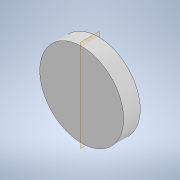
# Autodesk Inventor part: capFor6inchSch40Pipe
Saved by Autodesk Inventor 2021.1 (Build 251245000, 245)
## iProperties
Created: 2020-09-22
Part Number: capFor6inchSch40Pipe
Material: Generic
Document SubType Name: Modeling
Designer: robst
Density: 1 g/cm^3
Appearance: Default
Author: robst
Autodesk Inventor part; units mm, degrees
ref_plane "XZ Plane" through (0, 0, 0) normal (0, 1, 0) x (-1, 0, 0)
ref_plane "XY Plane" through (0, 0, 0) normal (0, 0, 1) x (1, 0, 0)
sketch "Sketch1" plane through (0, 0, 0) normal (0, 0, 1) x (1, 0, 0)
  circle A0 centre (0, 0) radius 87.3125
  circle A1 centre (0, 0) radius 92.075
  dimension "d0" = 174.625
  dimension "d1" = 4.7625
  constraints: 2 centre point, 2 coincident
  measures "d0" diameter of A0
  measures "d1" radial gap between concentric circles of A1 A0
extrude "Extrusion1" add sketch "Sketch1" along normal blind 4.7625 contours A0 | A1
extrude "Extrusion2" add sketch "Sketch1" against normal blind 31.75
sketch "Sketch2" plane through (0, 0, 0) normal (0, 0, -1) x (-1, 0, 0)
  line L0 (-80.4209, 0) -> (87.3125, 0) construction
  circle A0 centre (0, 0) radius 87.3125 construction
  spline S0 degree 2 poles (-73.9352, 1.1002) (-74.8615, 1.1002) (-76.4284, 1.7254) (-76.9996, 2.3506) knots 0 0 0 1 2 2 2
  spline S1 degree 2 poles (-76.9996, 2.3506) (-77.5708, 2.9681) (-78.196, 4.8206) (-78.196, 6.0248) knots 0 0 0 1 2 2 2
  spline S2 degree 2 poles (-78.196, 6.0248) (-78.196, 7.2212) (-77.5862, 8.9965) (-77.0073, 9.6526) knots 0 0 0 1 2 2 2
  spline S3 degree 2 poles (-77.0073, 9.6526) (-76.4361, 10.2933) (-74.8769, 10.9648) (-73.912, 10.9648) knots 0 0 0 1 2 2 2
  spline S4 degree 2 poles (-73.912, 10.9648) (-73.4335, 10.9648) (-72.5921, 10.8259) (-72.2371, 10.7178) knots 0 0 0 1 2 2 2
  spline S5 degree 2 poles (-72.2371, 10.7178) (-71.9283, 10.6175) (-71.2876, 10.3319) (-70.9712, 10.1621) knots 0 0 0 1 2 2 2
  line L1 (-70.9712, 10.1621) -> (-70.9712, 8.6337)
  line L2 (-70.9712, 8.6337) -> (-71.0715, 8.6337)
  spline S6 degree 2 poles (-71.0715, 8.6337) (-71.2413, 8.7881) (-71.7662, 9.2204) (-72.1444, 9.4288) knots 0 0 0 1 2 2 2
  spline S7 degree 2 poles (-72.1444, 9.4288) (-72.5072, 9.6295) (-73.364, 9.8842) (-73.9198, 9.8842) knots 0 0 0 1 2 2 2
  spline S8 degree 2 poles (-73.9198, 9.8842) (-74.5295, 9.8842) (-75.6179, 9.3825) (-76.027, 8.9039) knots 0 0 0 1 2 2 2
  spline S9 degree 2 poles (-76.027, 8.9039) (-76.4284, 8.4176) (-76.8761, 6.9433) (-76.8761, 6.0248) knots 0 0 0 1 2 2 2
  spline S10 degree 2 poles (-76.8761, 6.0248) (-76.8761, 5.0445) (-76.4052, 3.632) (-75.9961, 3.1457) knots 0 0 0 1 2 2 2
  spline S11 degree 2 poles (-75.9961, 3.1457) (-75.5947, 2.6748) (-74.5218, 2.1963) (-73.9198, 2.1963) knots 0 0 0 1 2 2 2
  spline S12 degree 2 poles (-73.9198, 2.1963) (-73.3717, 2.1963) (-72.4377, 2.4664) (-72.075, 2.6671) knots 0 0 0 1 2 2 2
  spline S13 degree 2 poles (-72.075, 2.6671) (-71.7276, 2.8678) (-71.2105, 3.2846) (-71.0638, 3.4313) knots 0 0 0 1 2 2 2
  line L3 (-71.0638, 3.4313) -> (-70.9712, 3.4313)
  line L4 (-70.9712, 3.4313) -> (-70.9712, 1.9184)
  spline S14 degree 2 poles (-70.9712, 1.9184) (-71.2876, 1.7717) (-71.8434, 1.5016) (-72.2371, 1.3781) knots 0 0 0 1 2 2 2
  spline S15 degree 2 poles (-72.2371, 1.3781) (-72.6539, 1.2391) (-73.364, 1.1002) (-73.9352, 1.1002) knots 0 0 0 1 2 2 2
  spline S16 degree 2 poles (-65.8999, 2.0264) (-66.0466, 1.9184) (-66.5406, 1.5324) (-66.7721, 1.4167) knots 0 0 0 1 2 2 2
  spline S17 degree 2 poles (-66.7721, 1.4167) (-67.0886, 1.2468) (-67.683, 1.0693) (-68.2233, 1.0693) knots 0 0 0 1 2 2 2
  spline S18 degree 2 poles (-68.2233, 1.0693) (-68.6633, 1.0693) (-69.4583, 1.4012) (-69.7593, 1.7023) knots 0 0 0 1 2 2 2
  spline S19 degree 2 poles (-69.7593, 1.7023) (-70.0449, 1.9956) (-70.3923, 2.8601) (-70.3923, 3.3386) knots 0 0 0 1 2 2 2
  spline S20 degree 2 poles (-70.3923, 3.3386) (-70.3923, 4.0796) (-69.767, 5.1294) (-69.0878, 5.4304) knots 0 0 0 1 2 2 2
  spline S21 degree 2 poles (-69.0878, 5.4304) (-68.4857, 5.7083) (-66.8493, 5.9167) (-65.8999, 5.9707) knots 0 0 0 1 2 2 2
  line L5 (-65.8999, 5.9707) -> (-65.8999, 6.2023)
  spline S22 degree 2 poles (-65.8999, 6.2023) (-65.8999, 6.6191) (-66.1546, 7.1363) (-66.3862, 7.2829) knots 0 0 0 1 2 2 2
  spline S23 degree 2 poles (-66.3862, 7.2829) (-66.6178, 7.4296) (-67.2816, 7.5222) (-67.6367, 7.5222) knots 0 0 0 1 2 2 2
  spline S24 degree 2 poles (-67.6367, 7.5222) (-68.0535, 7.5222) (-69.1804, 7.2752) (-69.7439, 7.0359) knots 0 0 0 1 2 2 2
  line L6 (-69.7439, 7.0359) -> (-69.8134, 7.0359)
  line L7 (-69.8134, 7.0359) -> (-69.8134, 8.2632)
  spline S25 degree 2 poles (-69.8134, 8.2632) (-69.4814, 8.3559) (-68.2387, 8.5874) (-67.6289, 8.5874) knots 0 0 0 1 2 2 2
  spline S26 degree 2 poles (-67.6289, 8.5874) (-66.8879, 8.5874) (-65.8768, 8.3559) (-65.4754, 8.0548) knots 0 0 0 1 2 2 2
  spline S27 degree 2 poles (-65.4754, 8.0548) (-65.0817, 7.7615) (-64.6958, 6.8275) (-64.6958, 6.156) knots 0 0 0 1 2 2 2
  line L8 (-64.6958, 6.156) -> (-64.6958, 1.27)
  line L9 (-64.6958, 1.27) -> (-65.8999, 1.27)
  line L10 (-65.8999, 1.27) -> (-65.8999, 2.0264)
  line L11 (-65.8999, 3.0299) -> (-65.8999, 5.0136)
  spline S28 degree 2 poles (-65.8999, 5.0136) (-66.3322, 4.975) (-67.6367, 4.8438) (-68.0458, 4.7203) knots 0 0 0 1 2 2 2
  spline S29 degree 2 poles (-68.0458, 4.7203) (-68.5243, 4.5736) (-69.1495, 3.9639) (-69.1495, 3.4235) knots 0 0 0 1 2 2 2
  spline S30 degree 2 poles (-69.1495, 3.4235) (-69.1495, 2.806) (-68.4548, 2.1808) (-67.791, 2.1808) knots 0 0 0 1 2 2 2
  spline S31 degree 2 poles (-67.791, 2.1808) (-67.2276, 2.1808) (-66.3013, 2.6671) (-65.8999, 3.0299) knots 0 0 0 1 2 2 2
  spline S32 degree 2 poles (-57.0156, 5.0368) (-57.0156, 3.246) (-58.7214, 1.1311) (-60.0259, 1.1311) knots 0 0 0 1 2 2 2
  spline S33 degree 2 poles (-60.0259, 1.1311) (-60.5585, 1.1311) (-61.3767, 1.3781) (-61.8012, 1.6328) knots 0 0 0 1 2 2 2
  line L12 (-61.8012, 1.6328) -> (-61.8012, -1.3621)
  line L13 (-61.8012, -1.3621) -> (-63.0054, -1.3621)
  line L14 (-63.0054, -1.3621) -> (-63.0054, 8.4176)
  line L15 (-63.0054, 8.4176) -> (-61.8012, 8.4176)
  line L16 (-61.8012, 8.4176) -> (-61.8012, 7.6689)
  spline S34 degree 2 poles (-61.8012, 7.6689) (-61.3536, 8.078) (-60.2575, 8.6183) (-59.6168, 8.6183) knots 0 0 0 1 2 2 2
  spline S35 degree 2 poles (-59.6168, 8.6183) (-58.3895, 8.6183) (-57.0156, 6.6732) (-57.0156, 5.0368) knots 0 0 0 1 2 2 2
  spline S36 degree 2 poles (-58.2583, 4.8978) (-58.2583, 6.1251) (-59.0379, 7.4759) (-59.9101, 7.4759) knots 0 0 0 1 2 2 2
  spline S37 degree 2 poles (-59.9101, 7.4759) (-60.4196, 7.4759) (-61.3767, 7.0205) (-61.8012, 6.6654) knots 0 0 0 1 2 2 2
  line L17 (-61.8012, 6.6654) -> (-61.8012, 2.6054)
  spline S38 degree 2 poles (-61.8012, 2.6054) (-61.3304, 2.3815) (-60.6589, 2.2117) (-60.2266, 2.2117) knots 0 0 0 1 2 2 2
  spline S39 degree 2 poles (-60.2266, 2.2117) (-59.2926, 2.2117) (-58.2583, 3.5856) (-58.2583, 4.8978) knots 0 0 0 1 2 2 2
  line L18 (-45.8851, 9.6681) -> (-50.3157, 9.6681)
  line L19 (-50.3157, 9.6681) -> (-50.3157, 6.9819)
  line L20 (-50.3157, 6.9819) -> (-46.0703, 6.9819)
  line L21 (-46.0703, 6.9819) -> (-46.0703, 5.855)
  line L22 (-46.0703, 5.855) -> (-50.3157, 5.855)
  line L23 (-50.3157, 5.855) -> (-50.3157, 1.27)
  line L24 (-50.3157, 1.27) -> (-51.5816, 1.27)
  line L25 (-51.5816, 1.27) -> (-51.5816, 10.795)
  line L26 (-51.5816, 10.795) -> (-45.8851, 10.795)
  line L27 (-45.8851, 10.795) -> (-45.8851, 9.6681)
  spline S40 degree 2 poles (-38.969, 4.8438) (-38.969, 3.0376) (-40.7058, 1.0693) (-42.1569, 1.0693) knots 0 0 0 1 2 2 2
  spline S41 degree 2 poles (-42.1569, 1.0693) (-43.6466, 1.0693) (-45.3525, 3.0994) (-45.3525, 4.8438) knots 0 0 0 1 2 2 2
  spline S42 degree 2 poles (-45.3525, 4.8438) (-45.3525, 6.6346) (-43.5926, 8.6183) (-42.1569, 8.6183) knots 0 0 0 1 2 2 2
  spline S43 degree 2 poles (-42.1569, 8.6183) (-40.7058, 8.6183) (-38.969, 6.6423) (-38.969, 4.8438) knots 0 0 0 1 2 2 2
  spline S44 degree 2 poles (-40.2118, 4.8438) (-40.2118, 6.2332) (-41.2229, 7.584) (-42.1569, 7.584) knots 0 0 0 1 2 2 2
  spline S45 degree 2 poles (-42.1569, 7.584) (-43.0909, 7.584) (-44.1098, 6.2332) (-44.1098, 4.8438) knots 0 0 0 1 2 2 2
  spline S46 degree 2 poles (-44.1098, 4.8438) (-44.1098, 3.493) (-43.0909, 2.1036) (-42.1569, 2.1036) knots 0 0 0 1 2 2 2
  spline S47 degree 2 poles (-42.1569, 2.1036) (-41.2306, 2.1036) (-40.2118, 3.4699) (-40.2118, 4.8438) knots 0 0 0 1 2 2 2
  line L28 (-33.9441, 7.1286) -> (-34.0058, 7.1286)
  spline S48 degree 2 poles (-34.0058, 7.1286) (-34.1448, 7.1672) (-34.4458, 7.1826) (-34.6542, 7.1826) knots 0 0 0 1 2 2 2
  spline S49 degree 2 poles (-34.6542, 7.1826) (-35.1405, 7.1826) (-36.0976, 6.7581) (-36.5299, 6.3413) knots 0 0 0 1 2 2 2
  line L29 (-36.5299, 6.3413) -> (-36.5299, 1.27)
  line L30 (-36.5299, 1.27) -> (-37.734, 1.27)
  line L31 (-37.734, 1.27) -> (-37.734, 8.4176)
  line L32 (-37.734, 8.4176) -> (-36.5299, 8.4176)
  line L33 (-36.5299, 8.4176) -> (-36.5299, 7.3524)
  spline S50 degree 2 poles (-36.5299, 7.3524) (-35.8738, 7.939) (-34.8935, 8.4176) (-34.4304, 8.4176) knots 0 0 0 1 2 2 2
  spline S51 degree 2 poles (-34.4304, 8.4176) (-34.2451, 8.4176) (-34.0599, 8.4022) (-33.9441, 8.379) knots 0 0 0 1 2 2 2
  line L34 (-33.9441, 8.379) -> (-33.9441, 7.1286)
  spline S52 degree 2 poles (-23.076, 4.3575) (-23.076, 3.6242) (-23.5623, 2.3815) (-23.9714, 1.9647) knots 0 0 0 1 2 2 2
  spline S53 degree 2 poles (-23.9714, 1.9647) (-24.3959, 1.5247) (-25.4611, 1.0693) (-26.1018, 1.0693) knots 0 0 0 1 2 2 2
  spline S54 degree 2 poles (-26.1018, 1.0693) (-26.7425, 1.0693) (-27.7999, 1.5016) (-28.2013, 1.9338) knots 0 0 0 1 2 2 2
  spline S55 degree 2 poles (-28.2013, 1.9338) (-28.6953, 2.451) (-29.2511, 4.1877) (-29.2511, 5.4536) knots 0 0 0 1 2 2 2
  spline S56 degree 2 poles (-29.2511, 5.4536) (-29.2511, 6.6963) (-28.7416, 8.6955) (-28.209, 9.4365) knots 0 0 0 1 2 2 2
  spline S57 degree 2 poles (-28.209, 9.4365) (-27.6919, 10.1621) (-26.0555, 10.9725) (-24.9826, 10.9725) knots 0 0 0 1 2 2 2
  spline S58 degree 2 poles (-24.9826, 10.9725) (-24.6661, 10.9725) (-24.1103, 10.9108) (-23.9019, 10.8413) knots 0 0 0 1 2 2 2
  line L35 (-23.9019, 10.8413) -> (-23.9019, 9.614)
  line L36 (-23.9019, 9.614) -> (-23.956, 9.614)
  spline S59 degree 2 poles (-23.956, 9.614) (-24.1335, 9.7066) (-24.7819, 9.8687) (-25.1524, 9.8687) knots 0 0 0 1 2 2 2
  spline S60 degree 2 poles (-25.1524, 9.8687) (-26.3411, 9.8687) (-27.7999, 8.2632) (-27.9389, 6.6886) knots 0 0 0 1 2 2 2
  spline S61 degree 2 poles (-27.9389, 6.6886) (-27.4835, 7.0051) (-26.5263, 7.3524) (-25.9551, 7.3524) knots 0 0 0 1 2 2 2
  spline S62 degree 2 poles (-25.9551, 7.3524) (-25.3994, 7.3524) (-24.5657, 7.1286) (-24.1103, 6.7889) knots 0 0 0 1 2 2 2
  spline S63 degree 2 poles (-24.1103, 6.7889) (-23.5855, 6.3953) (-23.076, 5.1757) (-23.076, 4.3575) knots 0 0 0 1 2 2 2
  spline S64 degree 2 poles (-24.3728, 4.3035) (-24.3728, 4.8901) (-24.6815, 5.6852) (-25.0212, 5.963) knots 0 0 0 1 2 2 2
  spline S65 degree 2 poles (-25.0212, 5.963) (-25.2759, 6.1637) (-25.9088, 6.2949) (-26.2407, 6.2949) knots 0 0 0 1 2 2 2
  spline S66 degree 2 poles (-26.2407, 6.2949) (-26.6884, 6.2949) (-27.5298, 6.0248) (-27.9389, 5.7701) knots 0 0 0 1 2 2 2
  spline S67 degree 2 poles (-27.9389, 5.7701) (-27.9466, 5.6311) (-27.962, 5.3687) (-27.962, 5.168) knots 0 0 0 1 2 2 2
  spline S68 degree 2 poles (-27.962, 5.168) (-27.962, 4.18) (-27.5761, 2.9681) (-27.2828, 2.6517) knots 0 0 0 1 2 2 2
  spline S69 degree 2 poles (-27.2828, 2.6517) (-27.0126, 2.3506) (-26.426, 2.1113) (-26.0941, 2.1113) knots 0 0 0 1 2 2 2
  spline S70 degree 2 poles (-26.0941, 2.1113) (-25.3222, 2.1113) (-24.3728, 3.2074) (-24.3728, 4.3035) knots 0 0 0 1 2 2 2
  line L37 (-18.1128, 11.2195) -> (-18.3907, 7.5145)
  line L38 (-18.3907, 7.5145) -> (-19.2321, 7.5145)
  line L39 (-19.2321, 7.5145) -> (-19.5099, 11.2195)
  line L40 (-19.5099, 11.2195) -> (-18.1128, 11.2195)
  line L41 (-20.5211, 11.2195) -> (-20.799, 7.5145)
  line L42 (-20.799, 7.5145) -> (-21.6403, 7.5145)
  line L43 (-21.6403, 7.5145) -> (-21.9182, 11.2195)
  line L44 (-21.9182, 11.2195) -> (-20.5211, 11.2195)
  spline S71 degree 2 poles (-9.6762, 1.1002) (-10.7105, 1.1002) (-12.1616, 1.5324) (-12.8023, 1.8412) knots 0 0 0 1 2 2 2
  line L45 (-12.8023, 1.8412) -> (-12.8023, 3.4313)
  line L46 (-12.8023, 3.4313) -> (-12.7097, 3.4313)
  spline S72 degree 2 poles (-12.7097, 3.4313) (-12.0844, 2.8446) (-10.5021, 2.1963) (-9.7688, 2.1963) knots 0 0 0 1 2 2 2
  spline S73 degree 2 poles (-9.7688, 2.1963) (-8.7191, 2.1963) (-7.6461, 3.0685) (-7.6461, 3.7863) knots 0 0 0 1 2 2 2
  spline S74 degree 2 poles (-7.6461, 3.7863) (-7.6461, 4.3575) (-8.2096, 5.0676) (-8.8194, 5.2452) knots 0 0 0 1 2 2 2
  spline S75 degree 2 poles (-8.8194, 5.2452) (-9.2594, 5.3687) (-9.9927, 5.5385) (-10.5407, 5.6774) knots 0 0 0 1 2 2 2
  spline S76 degree 2 poles (-10.5407, 5.6774) (-11.0347, 5.8087) (-11.8143, 6.2023) (-12.1153, 6.5188) knots 0 0 0 1 2 2 2
  spline S77 degree 2 poles (-12.1153, 6.5188) (-12.4086, 6.8353) (-12.7328, 7.6843) (-12.7328, 8.2401) knots 0 0 0 1 2 2 2
  spline S78 degree 2 poles (-12.7328, 8.2401) (-12.7328, 9.3979) (-10.9266, 10.9648) (-9.5295, 10.9648) knots 0 0 0 1 2 2 2
  spline S79 degree 2 poles (-9.5295, 10.9648) (-8.7268, 10.9648) (-7.3065, 10.6483) (-6.6967, 10.3473) knots 0 0 0 1 2 2 2
  line L47 (-6.6967, 10.3473) -> (-6.6967, 8.8344)
  line L48 (-6.6967, 8.8344) -> (-6.7894, 8.8344)
  spline S80 degree 2 poles (-6.7894, 8.8344) (-7.2448, 9.2512) (-8.665, 9.8687) (-9.4446, 9.8687) knots 0 0 0 1 2 2 2
  spline S81 degree 2 poles (-9.4446, 9.8687) (-10.3246, 9.8687) (-11.4129, 9.0428) (-11.4129, 8.3713) knots 0 0 0 1 2 2 2
  spline S82 degree 2 poles (-11.4129, 8.3713) (-11.4129, 7.7692) (-10.7723, 7.0514) (-10.1702, 6.8893) knots 0 0 0 1 2 2 2
  spline S83 degree 2 poles (-10.1702, 6.8893) (-9.7688, 6.7812) (-8.6033, 6.5033) (-8.2173, 6.3876) knots 0 0 0 1 2 2 2
  spline S84 degree 2 poles (-8.2173, 6.3876) (-7.237, 6.0865) (-6.3262, 4.8747) (-6.3262, 3.987) knots 0 0 0 1 2 2 2
  spline S85 degree 2 poles (-6.3262, 3.987) (-6.3262, 3.4235) (-6.7816, 2.3429) (-7.1907, 1.9647) knots 0 0 0 1 2 2 2
  spline S86 degree 2 poles (-7.1907, 1.9647) (-7.6461, 1.5479) (-8.804, 1.1002) (-9.6762, 1.1002) knots 0 0 0 1 2 2 2
  spline S87 degree 2 poles (-2.2893, 1.1079) (-3.0303, 1.1079) (-4.2576, 1.5633) (-4.6976, 2.0264) knots 0 0 0 1 2 2 2
  spline S88 degree 2 poles (-4.6976, 2.0264) (-5.1375, 2.4819) (-5.6238, 3.8867) (-5.6238, 4.8284) knots 0 0 0 1 2 2 2
  spline S89 degree 2 poles (-5.6238, 4.8284) (-5.6238, 5.7701) (-5.1221, 7.144) (-4.6976, 7.6071) knots 0 0 0 1 2 2 2
  spline S90 degree 2 poles (-4.6976, 7.6071) (-4.273, 8.078) (-3.0149, 8.5797) (-2.2893, 8.5797) knots 0 0 0 1 2 2 2
  spline S91 degree 2 poles (-2.2893, 8.5797) (-1.7027, 8.5797) (-0.6066, 8.2478) (-0.1821, 8.0317) knots 0 0 0 1 2 2 2
  line L49 (-0.1821, 8.0317) -> (-0.1821, 6.6809)
  line L50 (-0.1821, 6.6809) -> (-0.2515, 6.6809)
  spline S92 degree 2 poles (-0.2515, 6.6809) (-0.3827, 6.7889) (-0.7841, 7.0668) (-1.0697, 7.2135) knots 0 0 0 1 2 2 2
  spline S93 degree 2 poles (-1.0697, 7.2135) (-1.3244, 7.337) (-2.0037, 7.5299) (-2.3124, 7.5299) knots 0 0 0 1 2 2 2
  spline S94 degree 2 poles (-2.3124, 7.5299) (-3.2464, 7.5299) (-4.3811, 6.1174) (-4.3811, 4.8284) knots 0 0 0 1 2 2 2
  spline S95 degree 2 poles (-4.3811, 4.8284) (-4.3811, 3.5702) (-3.285, 2.1577) (-2.3124, 2.1577) knots 0 0 0 1 2 2 2
  spline S96 degree 2 poles (-2.3124, 2.1577) (-1.7258, 2.1577) (-0.6606, 2.6439) (-0.2515, 3.0222) knots 0 0 0 1 2 2 2
  line L51 (-0.2515, 3.0222) -> (-0.1821, 3.0222)
  line L52 (-0.1821, 3.0222) -> (-0.1821, 1.6714)
  spline S97 degree 2 poles (-0.1821, 1.6714) (-0.3596, 1.5865) (-0.8999, 1.3472) (-1.116, 1.2932) knots 0 0 0 1 2 2 2
  spline S98 degree 2 poles (-1.116, 1.2932) (-1.4248, 1.2005) (-1.9111, 1.1079) (-2.2893, 1.1079) knots 0 0 0 1 2 2 2
  line L53 (6.5256, 1.27) -> (5.3214, 1.27)
  line L54 (5.3214, 1.27) -> (5.3214, 5.3455)
  spline S99 degree 2 poles (5.3214, 5.3455) (5.3214, 5.8395) (5.2288, 6.6886) (5.0899, 6.9433) knots 0 0 0 1 2 2 2
  spline S100 degree 2 poles (5.0899, 6.9433) (4.9432, 7.2135) (4.4183, 7.4759) (3.9707, 7.4759) knots 0 0 0 1 2 2 2
  spline S101 degree 2 poles (3.9707, 7.4759) (3.523, 7.4759) (2.5736, 6.9973) (2.1181, 6.6114) knots 0 0 0 1 2 2 2
  line L55 (2.1181, 6.6114) -> (2.1181, 1.27)
  line L56 (2.1181, 1.27) -> (0.914, 1.27)
  line L57 (0.914, 1.27) -> (0.914, 11.2195)
  line L58 (0.914, 11.2195) -> (2.1181, 11.2195)
  line L59 (2.1181, 11.2195) -> (2.1181, 7.6226)
  spline S102 degree 2 poles (2.1181, 7.6226) (2.6585, 8.1089) (3.7005, 8.6183) (4.2871, 8.6183) knots 0 0 0 1 2 2 2
  spline S103 degree 2 poles (4.2871, 8.6183) (5.3369, 8.6183) (6.5256, 7.2289) (6.5256, 5.909) knots 0 0 0 1 2 2 2
  line L60 (6.5256, 5.909) -> (6.5256, 1.27)
  spline S104 degree 2 poles (11.319, 1.1079) (9.6054, 1.1079) (7.722, 3.0299) (7.722, 4.8052) knots 0 0 0 1 2 2 2
  spline S105 degree 2 poles (7.722, 4.8052) (7.722, 6.5497) (9.5513, 8.6183) (11.0256, 8.6183) knots 0 0 0 1 2 2 2
  spline S106 degree 2 poles (11.0256, 8.6183) (11.6895, 8.6183) (12.7161, 8.2324) (13.0943, 7.8233) knots 0 0 0 1 2 2 2
  spline S107 degree 2 poles (13.0943, 7.8233) (13.4802, 7.4142) (13.8893, 6.2332) (13.8893, 5.3764) knots 0 0 0 1 2 2 2
  line L61 (13.8893, 5.3764) -> (13.8893, 4.7203)
  line L62 (13.8893, 4.7203) -> (8.9416, 4.7203)
  spline S108 degree 2 poles (8.9416, 4.7203) (8.9416, 3.4776) (10.192, 2.1577) (11.3035, 2.1577) knots 0 0 0 1 2 2 2
  spline S109 degree 2 poles (11.3035, 2.1577) (11.6972, 2.1577) (12.4613, 2.3352) (12.7701, 2.4741) knots 0 0 0 1 2 2 2
  spline S110 degree 2 poles (12.7701, 2.4741) (13.0943, 2.6285) (13.542, 2.8987) (13.6886, 3.0222) knots 0 0 0 1 2 2 2
  line L63 (13.6886, 3.0222) -> (13.7581, 3.0222)
  line L64 (13.7581, 3.0222) -> (13.7581, 1.71)
  spline S111 degree 2 poles (13.7581, 1.71) (13.5497, 1.6251) (12.9167, 1.3781) (12.6697, 1.3086) knots 0 0 0 1 2 2 2
  spline S112 degree 2 poles (12.6697, 1.3086) (12.3224, 1.2082) (11.7512, 1.1079) (11.319, 1.1079) knots 0 0 0 1 2 2 2
  spline S113 degree 2 poles (12.7161, 5.6388) (12.7006, 6.1251) (12.4999, 6.8353) (12.307, 7.0745) knots 0 0 0 1 2 2 2
  spline S114 degree 2 poles (12.307, 7.0745) (12.0986, 7.3447) (11.4425, 7.6303) (10.9562, 7.6303) knots 0 0 0 1 2 2 2
  spline S115 degree 2 poles (10.9562, 7.6303) (10.4776, 7.6303) (9.8061, 7.3447) (9.5282, 7.0668) knots 0 0 0 1 2 2 2
  spline S116 degree 2 poles (9.5282, 7.0668) (9.258, 6.7812) (8.9802, 6.0943) (8.9416, 5.6388) knots 0 0 0 1 2 2 2
  line L65 (8.9416, 5.6388) -> (12.7161, 5.6388)
  line L66 (20.6047, 1.27) -> (19.4005, 1.27)
  line L67 (19.4005, 1.27) -> (19.4005, 1.9956)
  spline S117 degree 2 poles (19.4005, 1.9956) (19.1227, 1.764) (18.7136, 1.4553) (18.4357, 1.324) knots 0 0 0 1 2 2 2
  spline S118 degree 2 poles (18.4357, 1.324) (18.181, 1.2005) (17.6329, 1.0693) (17.2701, 1.0693) knots 0 0 0 1 2 2 2
  spline S119 degree 2 poles (17.2701, 1.0693) (16.6835, 1.0693) (15.6955, 1.5556) (15.3482, 2.0264) knots 0 0 0 1 2 2 2
  spline S120 degree 2 poles (15.3482, 2.0264) (15.0008, 2.4973) (14.6149, 3.8867) (14.6149, 4.7898) knots 0 0 0 1 2 2 2
  spline S121 degree 2 poles (14.6149, 4.7898) (14.6149, 5.7315) (15.1012, 7.1054) (15.5257, 7.6226) knots 0 0 0 1 2 2 2
  spline S122 degree 2 poles (15.5257, 7.6226) (15.9194, 8.0857) (17.0231, 8.6183) (17.6329, 8.6183) knots 0 0 0 1 2 2 2
  spline S123 degree 2 poles (17.6329, 8.6183) (18.1655, 8.6183) (18.9606, 8.379) (19.4005, 8.132) knots 0 0 0 1 2 2 2
  line L68 (19.4005, 8.132) -> (19.4005, 11.2195)
  line L69 (19.4005, 11.2195) -> (20.6047, 11.2195)
  line L70 (20.6047, 11.2195) -> (20.6047, 1.27)
  line L71 (19.4005, 3.0067) -> (19.4005, 7.1363)
  spline S124 degree 2 poles (19.4005, 7.1363) (18.9528, 7.3524) (18.2427, 7.5145) (17.8336, 7.5145) knots 0 0 0 1 2 2 2
  spline S125 degree 2 poles (17.8336, 7.5145) (16.9074, 7.5145) (15.8576, 6.1251) (15.8576, 4.8129) knots 0 0 0 1 2 2 2
  spline S126 degree 2 poles (15.8576, 4.8129) (15.8576, 3.547) (16.6604, 2.2117) (17.548, 2.2117) knots 0 0 0 1 2 2 2
  spline S127 degree 2 poles (17.548, 2.2117) (18.0189, 2.2117) (18.976, 2.6439) (19.4005, 3.0067) knots 0 0 0 1 2 2 2
  line L72 (27.9067, 1.27) -> (26.7025, 1.27)
  line L73 (26.7025, 1.27) -> (26.7025, 2.0573)
  spline S128 degree 2 poles (26.7025, 2.0573) (26.1468, 1.571) (25.151, 1.0693) (24.5335, 1.0693) knots 0 0 0 1 2 2 2
  spline S129 degree 2 poles (24.5335, 1.0693) (24.0704, 1.0693) (23.2445, 1.3781) (22.9435, 1.71) knots 0 0 0 1 2 2 2
  spline S130 degree 2 poles (22.9435, 1.71) (22.6347, 2.0419) (22.2951, 3.053) (22.2951, 3.7786) knots 0 0 0 1 2 2 2
  line L74 (22.2951, 3.7786) -> (22.2951, 8.4176)
  line L75 (22.2951, 8.4176) -> (23.4992, 8.4176)
  line L76 (23.4992, 8.4176) -> (23.4992, 4.3421)
  spline S131 degree 2 poles (23.4992, 4.3421) (23.4992, 3.7709) (23.5841, 3.0222) (23.7308, 2.7443) knots 0 0 0 1 2 2 2
  spline S132 degree 2 poles (23.7308, 2.7443) (23.8774, 2.4664) (24.3792, 2.2117) (24.85, 2.2117) knots 0 0 0 1 2 2 2
  spline S133 degree 2 poles (24.85, 2.2117) (25.29, 2.2117) (26.2857, 2.7134) (26.7025, 3.0762) knots 0 0 0 1 2 2 2
  line L77 (26.7025, 3.0762) -> (26.7025, 8.4176)
  line L78 (26.7025, 8.4176) -> (27.9067, 8.4176)
  line L79 (27.9067, 8.4176) -> (27.9067, 1.27)
  line L80 (30.8784, 1.27) -> (29.6743, 1.27)
  line L81 (29.6743, 1.27) -> (29.6743, 11.2195)
  line L82 (29.6743, 11.2195) -> (30.8784, 11.2195)
  line L83 (30.8784, 11.2195) -> (30.8784, 1.27)
  spline S134 degree 2 poles (35.749, 1.1079) (34.0354, 1.1079) (32.152, 3.0299) (32.152, 4.8052) knots 0 0 0 1 2 2 2
  spline S135 degree 2 poles (32.152, 4.8052) (32.152, 6.5497) (33.9814, 8.6183) (35.4556, 8.6183) knots 0 0 0 1 2 2 2
  spline S136 degree 2 poles (35.4556, 8.6183) (36.1195, 8.6183) (37.1461, 8.2324) (37.5243, 7.8233) knots 0 0 0 1 2 2 2
  spline S137 degree 2 poles (37.5243, 7.8233) (37.9102, 7.4142) (38.3193, 6.2332) (38.3193, 5.3764) knots 0 0 0 1 2 2 2
  line L84 (38.3193, 5.3764) -> (38.3193, 4.7203)
  line L85 (38.3193, 4.7203) -> (33.3716, 4.7203)
  spline S138 degree 2 poles (33.3716, 4.7203) (33.3716, 3.4776) (34.622, 2.1577) (35.7335, 2.1577) knots 0 0 0 1 2 2 2
  spline S139 degree 2 poles (35.7335, 2.1577) (36.1272, 2.1577) (36.8913, 2.3352) (37.2001, 2.4741) knots 0 0 0 1 2 2 2
  spline S140 degree 2 poles (37.2001, 2.4741) (37.5243, 2.6285) (37.972, 2.8987) (38.1186, 3.0222) knots 0 0 0 1 2 2 2
  line L86 (38.1186, 3.0222) -> (38.1881, 3.0222)
  line L87 (38.1881, 3.0222) -> (38.1881, 1.71)
  spline S141 degree 2 poles (38.1881, 1.71) (37.9797, 1.6251) (37.3467, 1.3781) (37.0997, 1.3086) knots 0 0 0 1 2 2 2
  spline S142 degree 2 poles (37.0997, 1.3086) (36.7524, 1.2082) (36.1812, 1.1079) (35.749, 1.1079) knots 0 0 0 1 2 2 2
  spline S143 degree 2 poles (37.1461, 5.6388) (37.1306, 6.1251) (36.9299, 6.8353) (36.737, 7.0745) knots 0 0 0 1 2 2 2
  spline S144 degree 2 poles (36.737, 7.0745) (36.5286, 7.3447) (35.8725, 7.6303) (35.3862, 7.6303) knots 0 0 0 1 2 2 2
  spline S145 degree 2 poles (35.3862, 7.6303) (34.9076, 7.6303) (34.2361, 7.3447) (33.9582, 7.0668) knots 0 0 0 1 2 2 2
  spline S146 degree 2 poles (33.9582, 7.0668) (33.688, 6.7812) (33.4102, 6.0943) (33.3716, 5.6388) knots 0 0 0 1 2 2 2
  line L88 (33.3716, 5.6388) -> (37.1461, 5.6388)
  line L89 (49.581, 4.5428) -> (48.4464, 4.5428)
  line L90 (48.4464, 4.5428) -> (48.4464, 1.27)
  line L91 (48.4464, 1.27) -> (47.2191, 1.27)
  line L92 (47.2191, 1.27) -> (47.2191, 4.5428)
  line L93 (47.2191, 4.5428) -> (43.0123, 4.5428)
  line L94 (43.0123, 4.5428) -> (43.0123, 5.8858)
  line L95 (43.0123, 5.8858) -> (47.2731, 10.795)
  line L96 (47.2731, 10.795) -> (48.4464, 10.795)
  line L97 (48.4464, 10.795) -> (48.4464, 5.5694)
  line L98 (48.4464, 5.5694) -> (49.581, 5.5694)
  line L99 (49.581, 5.5694) -> (49.581, 4.5428)
  line L100 (47.2191, 5.5694) -> (47.2191, 9.2898)
  line L101 (47.2191, 9.2898) -> (44.0158, 5.5694)
  line L102 (44.0158, 5.5694) -> (47.2191, 5.5694)
  spline S147 degree 2 poles (56.528, 6.0325) (56.528, 3.4699) (55.0382, 1.0693) (53.4868, 1.0693) knots 0 0 0 1 2 2 2
  spline S148 degree 2 poles (53.4868, 1.0693) (51.9121, 1.0693) (50.4378, 3.5162) (50.4378, 6.0248) knots 0 0 0 1 2 2 2
  spline S149 degree 2 poles (50.4378, 6.0248) (50.4378, 8.6029) (51.9276, 10.988) (53.4868, 10.988) knots 0 0 0 1 2 2 2
  spline S150 degree 2 poles (53.4868, 10.988) (55.0537, 10.988) (56.528, 8.518) (56.528, 6.0325) knots 0 0 0 1 2 2 2
  spline S151 degree 2 poles (54.8916, 3.1302) (55.0768, 3.6011) (55.2312, 5.0522) (55.2312, 6.0325) knots 0 0 0 1 2 2 2
  spline S152 degree 2 poles (55.2312, 6.0325) (55.2312, 7.0128) (55.0768, 8.4562) (54.8839, 8.9425) knots 0 0 0 1 2 2 2
  spline S153 degree 2 poles (54.8839, 8.9425) (54.6909, 9.4288) (54.0194, 9.9305) (53.4868, 9.9305) knots 0 0 0 1 2 2 2
  spline S154 degree 2 poles (53.4868, 9.9305) (52.9542, 9.9305) (52.2672, 9.4288) (52.0665, 8.9271) knots 0 0 0 1 2 2 2
  spline S155 degree 2 poles (52.0665, 8.9271) (51.8735, 8.4408) (51.7346, 6.9588) (51.7346, 6.0248) knots 0 0 0 1 2 2 2
  spline S156 degree 2 poles (51.7346, 6.0248) (51.7346, 5.0213) (51.8581, 3.6783) (52.0588, 3.1534) knots 0 0 0 1 2 2 2
  spline S157 degree 2 poles (52.0588, 3.1534) (52.244, 2.6594) (52.931, 2.1268) (53.4868, 2.1268) knots 0 0 0 1 2 2 2
  spline S158 degree 2 poles (53.4868, 2.1268) (54.0116, 2.1268) (54.6986, 2.6285) (54.8916, 3.1302) knots 0 0 0 1 2 2 2
  spline S159 degree 2 poles (68.0058, 5.0368) (68.0058, 3.246) (66.3, 1.1311) (64.9955, 1.1311) knots 0 0 0 1 2 2 2
  spline S160 degree 2 poles (64.9955, 1.1311) (64.4629, 1.1311) (63.6447, 1.3781) (63.2202, 1.6328) knots 0 0 0 1 2 2 2
  line L103 (63.2202, 1.6328) -> (63.2202, -1.3621)
  line L104 (63.2202, -1.3621) -> (62.016, -1.3621)
  line L105 (62.016, -1.3621) -> (62.016, 8.4176)
  line L106 (62.016, 8.4176) -> (63.2202, 8.4176)
  line L107 (63.2202, 8.4176) -> (63.2202, 7.6689)
  spline S161 degree 2 poles (63.2202, 7.6689) (63.6679, 8.078) (64.7639, 8.6183) (65.4046, 8.6183) knots 0 0 0 1 2 2 2
  spline S162 degree 2 poles (65.4046, 8.6183) (66.6319, 8.6183) (68.0058, 6.6732) (68.0058, 5.0368) knots 0 0 0 1 2 2 2
  spline S163 degree 2 poles (66.7631, 4.8978) (66.7631, 6.1251) (65.9835, 7.4759) (65.1113, 7.4759) knots 0 0 0 1 2 2 2
  spline S164 degree 2 poles (65.1113, 7.4759) (64.6018, 7.4759) (63.6447, 7.0205) (63.2202, 6.6654) knots 0 0 0 1 2 2 2
  line L108 (63.2202, 6.6654) -> (63.2202, 2.6054)
  spline S165 degree 2 poles (63.2202, 2.6054) (63.691, 2.3815) (64.3625, 2.2117) (64.7948, 2.2117) knots 0 0 0 1 2 2 2
  spline S166 degree 2 poles (64.7948, 2.2117) (65.7288, 2.2117) (66.7631, 3.5856) (66.7631, 4.8978) knots 0 0 0 1 2 2 2
  line L109 (70.4836, 1.27) -> (69.2794, 1.27)
  line L110 (69.2794, 1.27) -> (69.2794, 8.4176)
  line L111 (69.2794, 8.4176) -> (70.4836, 8.4176)
  line L112 (70.4836, 8.4176) -> (70.4836, 1.27)
  line L113 (70.5685, 9.6063) -> (69.2022, 9.6063)
  line L114 (69.2022, 9.6063) -> (69.2022, 10.8568)
  line L115 (69.2022, 10.8568) -> (70.5685, 10.8568)
  line L116 (70.5685, 10.8568) -> (70.5685, 9.6063)
  spline S167 degree 2 poles (78.241, 5.0368) (78.241, 3.246) (76.5351, 1.1311) (75.2306, 1.1311) knots 0 0 0 1 2 2 2
  spline S168 degree 2 poles (75.2306, 1.1311) (74.698, 1.1311) (73.8798, 1.3781) (73.4553, 1.6328) knots 0 0 0 1 2 2 2
  line L117 (73.4553, 1.6328) -> (73.4553, -1.3621)
  line L118 (73.4553, -1.3621) -> (72.2512, -1.3621)
  line L119 (72.2512, -1.3621) -> (72.2512, 8.4176)
  line L120 (72.2512, 8.4176) -> (73.4553, 8.4176)
  line L121 (73.4553, 8.4176) -> (73.4553, 7.6689)
  spline S169 degree 2 poles (73.4553, 7.6689) (73.903, 8.078) (74.9991, 8.6183) (75.6397, 8.6183) knots 0 0 0 1 2 2 2
  spline S170 degree 2 poles (75.6397, 8.6183) (76.867, 8.6183) (78.241, 6.6732) (78.241, 5.0368) knots 0 0 0 1 2 2 2
  spline S171 degree 2 poles (76.9982, 4.8978) (76.9982, 6.1251) (76.2186, 7.4759) (75.3464, 7.4759) knots 0 0 0 1 2 2 2
  spline S172 degree 2 poles (75.3464, 7.4759) (74.837, 7.4759) (73.8798, 7.0205) (73.4553, 6.6654) knots 0 0 0 1 2 2 2
  line L122 (73.4553, 6.6654) -> (73.4553, 2.6054)
  spline S173 degree 2 poles (73.4553, 2.6054) (73.9261, 2.3815) (74.5977, 2.2117) (75.0299, 2.2117) knots 0 0 0 1 2 2 2
  spline S174 degree 2 poles (75.0299, 2.2117) (75.9639, 2.2117) (76.9982, 3.5856) (76.9982, 4.8978) knots 0 0 0 1 2 2 2
  spline S175 degree 2 poles (82.5944, 1.1079) (80.8808, 1.1079) (78.9974, 3.0299) (78.9974, 4.8052) knots 0 0 0 1 2 2 2
  spline S176 degree 2 poles (78.9974, 4.8052) (78.9974, 6.5497) (80.8267, 8.6183) (82.301, 8.6183) knots 0 0 0 1 2 2 2
  spline S177 degree 2 poles (82.301, 8.6183) (82.9649, 8.6183) (83.9915, 8.2324) (84.3697, 7.8233) knots 0 0 0 1 2 2 2
  spline S178 degree 2 poles (84.3697, 7.8233) (84.7556, 7.4142) (85.1647, 6.2332) (85.1647, 5.3764) knots 0 0 0 1 2 2 2
  line L123 (85.1647, 5.3764) -> (85.1647, 4.7203)
  line L124 (85.1647, 4.7203) -> (80.217, 4.7203)
  spline S179 degree 2 poles (80.217, 4.7203) (80.217, 3.4776) (81.4674, 2.1577) (82.5789, 2.1577) knots 0 0 0 1 2 2 2
  spline S180 degree 2 poles (82.5789, 2.1577) (82.9726, 2.1577) (83.7367, 2.3352) (84.0455, 2.4741) knots 0 0 0 1 2 2 2
  spline S181 degree 2 poles (84.0455, 2.4741) (84.3697, 2.6285) (84.8174, 2.8987) (84.964, 3.0222) knots 0 0 0 1 2 2 2
  line L125 (84.964, 3.0222) -> (85.0335, 3.0222)
  line L126 (85.0335, 3.0222) -> (85.0335, 1.71)
  spline S182 degree 2 poles (85.0335, 1.71) (84.8251, 1.6251) (84.1921, 1.3781) (83.9451, 1.3086) knots 0 0 0 1 2 2 2
  spline S183 degree 2 poles (83.9451, 1.3086) (83.5978, 1.2082) (83.0266, 1.1079) (82.5944, 1.1079) knots 0 0 0 1 2 2 2
  spline S184 degree 2 poles (83.9915, 5.6388) (83.976, 6.1251) (83.7753, 6.8353) (83.5824, 7.0745) knots 0 0 0 1 2 2 2
  spline S185 degree 2 poles (83.5824, 7.0745) (83.374, 7.3447) (82.7179, 7.6303) (82.2316, 7.6303) knots 0 0 0 1 2 2 2
  spline S186 degree 2 poles (82.2316, 7.6303) (81.753, 7.6303) (81.0815, 7.3447) (80.8036, 7.0668) knots 0 0 0 1 2 2 2
  spline S187 degree 2 poles (80.8036, 7.0668) (80.5334, 6.7812) (80.2556, 6.0943) (80.217, 5.6388) knots 0 0 0 1 2 2 2
  line L127 (80.217, 5.6388) -> (83.9915, 5.6388)
  line L128 (-19.2166, -4.9342) -> (-22.4971, -14.4592)
  line L129 (-22.4971, -14.4592) -> (-23.8633, -14.4592)
  line L130 (-23.8633, -14.4592) -> (-27.1438, -4.9342)
  line L131 (-27.1438, -4.9342) -> (-25.7853, -4.9342)
  line L132 (-25.7853, -4.9342) -> (-23.1455, -12.846)
  line L133 (-23.1455, -12.846) -> (-20.5057, -4.9342)
  line L134 (-20.5057, -4.9342) -> (-19.2166, -4.9342)
  spline S188 degree 2 poles (-15.1874, -14.6213) (-16.901, -14.6213) (-18.7844, -12.6993) (-18.7844, -10.924) knots 0 0 0 1 2 2 2
  spline S189 degree 2 poles (-18.7844, -10.924) (-18.7844, -9.1795) (-16.955, -7.1109) (-15.4807, -7.1109) knots 0 0 0 1 2 2 2
  spline S190 degree 2 poles (-15.4807, -7.1109) (-14.8169, -7.1109) (-13.7903, -7.4968) (-13.4121, -7.9059) knots 0 0 0 1 2 2 2
  spline S191 degree 2 poles (-13.4121, -7.9059) (-13.0261, -8.315) (-12.617, -9.496) (-12.617, -10.3528) knots 0 0 0 1 2 2 2
  line L135 (-12.617, -10.3528) -> (-12.617, -11.0089)
  line L136 (-12.617, -11.0089) -> (-17.5648, -11.0089)
  spline S192 degree 2 poles (-17.5648, -11.0089) (-17.5648, -12.2516) (-16.3143, -13.5715) (-15.2028, -13.5715) knots 0 0 0 1 2 2 2
  spline S193 degree 2 poles (-15.2028, -13.5715) (-14.8092, -13.5715) (-14.045, -13.394) (-13.7363, -13.2551) knots 0 0 0 1 2 2 2
  spline S194 degree 2 poles (-13.7363, -13.2551) (-13.4121, -13.1007) (-12.9644, -12.8305) (-12.8177, -12.707) knots 0 0 0 1 2 2 2
  line L137 (-12.8177, -12.707) -> (-12.7483, -12.707)
  line L138 (-12.7483, -12.707) -> (-12.7483, -14.0192)
  spline S195 degree 2 poles (-12.7483, -14.0192) (-12.9567, -14.1041) (-13.5896, -14.3511) (-13.8366, -14.4206) knots 0 0 0 1 2 2 2
  spline S196 degree 2 poles (-13.8366, -14.4206) (-14.184, -14.5209) (-14.7552, -14.6213) (-15.1874, -14.6213) knots 0 0 0 1 2 2 2
  spline S197 degree 2 poles (-13.7903, -10.0904) (-13.8057, -9.6041) (-14.0064, -8.8939) (-14.1994, -8.6547) knots 0 0 0 1 2 2 2
  spline S198 degree 2 poles (-14.1994, -8.6547) (-14.4078, -8.3845) (-15.0639, -8.0989) (-15.5502, -8.0989) knots 0 0 0 1 2 2 2
  spline S199 degree 2 poles (-15.5502, -8.0989) (-16.0288, -8.0989) (-16.7003, -8.3845) (-16.9782, -8.6624) knots 0 0 0 1 2 2 2
  spline S200 degree 2 poles (-16.9782, -8.6624) (-17.2483, -8.948) (-17.5262, -9.6349) (-17.5648, -10.0904) knots 0 0 0 1 2 2 2
  line L139 (-17.5648, -10.0904) -> (-13.7903, -10.0904)
  line L140 (-7.6075, -8.6006) -> (-7.6693, -8.6006)
  spline S201 degree 2 poles (-7.6693, -8.6006) (-7.8082, -8.562) (-8.1093, -8.5466) (-8.3177, -8.5466) knots 0 0 0 1 2 2 2
  spline S202 degree 2 poles (-8.3177, -8.5466) (-8.804, -8.5466) (-9.7611, -8.9711) (-10.1933, -9.3879) knots 0 0 0 1 2 2 2
  line L141 (-10.1933, -9.3879) -> (-10.1933, -14.4592)
  line L142 (-10.1933, -14.4592) -> (-11.3975, -14.4592)
  line L143 (-11.3975, -14.4592) -> (-11.3975, -7.3116)
  line L144 (-11.3975, -7.3116) -> (-10.1933, -7.3116)
  line L145 (-10.1933, -7.3116) -> (-10.1933, -8.3768)
  spline S203 degree 2 poles (-10.1933, -8.3768) (-9.5372, -7.7902) (-8.557, -7.3116) (-8.0938, -7.3116) knots 0 0 0 1 2 2 2
  spline S204 degree 2 poles (-8.0938, -7.3116) (-7.9086, -7.3116) (-7.7233, -7.327) (-7.6075, -7.3502) knots 0 0 0 1 2 2 2
  line L146 (-7.6075, -7.3502) -> (-7.6075, -8.6006)
  spline S205 degree 2 poles (-4.7439, -14.629) (-5.4617, -14.629) (-6.7044, -14.2431) (-7.1135, -14.0269) knots 0 0 0 1 2 2 2
  line L147 (-7.1135, -14.0269) -> (-7.1135, -12.6762)
  line L148 (-7.1135, -12.6762) -> (-7.0518, -12.6762)
  spline S206 degree 2 poles (-7.0518, -12.6762) (-6.8974, -12.7997) (-6.4806, -13.093) (-6.1333, -13.2551) knots 0 0 0 1 2 2 2
  spline S207 degree 2 poles (-6.1333, -13.2551) (-5.8322, -13.4017) (-5.0912, -13.6178) (-4.6976, -13.6178) knots 0 0 0 1 2 2 2
  spline S208 degree 2 poles (-4.6976, -13.6178) (-4.412, -13.6178) (-3.7559, -13.4866) (-3.6015, -13.3786) knots 0 0 0 1 2 2 2
  spline S209 degree 2 poles (-3.6015, -13.3786) (-3.3776, -13.2319) (-3.177, -12.9) (-3.177, -12.5604) knots 0 0 0 1 2 2 2
  spline S210 degree 2 poles (-3.177, -12.5604) (-3.177, -12.1358) (-3.6401, -11.6959) (-4.2344, -11.5492) knots 0 0 0 1 2 2 2
  spline S211 degree 2 poles (-4.2344, -11.5492) (-4.466, -11.4952) (-5.207, -11.3408) (-5.5235, -11.2559) knots 0 0 0 1 2 2 2
  spline S212 degree 2 poles (-5.5235, -11.2559) (-6.3417, -11.0166) (-7.0827, -10.0286) (-7.0827, -9.3262) knots 0 0 0 1 2 2 2
  spline S213 degree 2 poles (-7.0827, -9.3262) (-7.0827, -8.3536) (-5.6238, -7.1418) (-4.4197, -7.1418) knots 0 0 0 1 2 2 2
  spline S214 degree 2 poles (-4.4197, -7.1418) (-3.8253, -7.1418) (-2.6212, -7.4351) (-2.2121, -7.6589) knots 0 0 0 1 2 2 2
  line L149 (-2.2121, -7.6589) -> (-2.2121, -8.948)
  line L150 (-2.2121, -8.948) -> (-2.2739, -8.948)
  spline S215 degree 2 poles (-2.2739, -8.948) (-2.737, -8.5775) (-3.8639, -8.1529) (-4.4428, -8.1529) knots 0 0 0 1 2 2 2
  spline S216 degree 2 poles (-4.4428, -8.1529) (-5.0372, -8.1529) (-5.8554, -8.6547) (-5.8554, -9.1564) knots 0 0 0 1 2 2 2
  spline S217 degree 2 poles (-5.8554, -9.1564) (-5.8554, -9.6118) (-5.3691, -10.0518) (-4.8288, -10.1907) knots 0 0 0 1 2 2 2
  spline S218 degree 2 poles (-4.8288, -10.1907) (-4.5663, -10.2602) (-3.9025, -10.3991) (-3.5397, -10.484) knots 0 0 0 1 2 2 2
  spline S219 degree 2 poles (-3.5397, -10.484) (-2.7524, -10.6847) (-1.9497, -11.6032) (-1.9497, -12.3983) knots 0 0 0 1 2 2 2
  spline S220 degree 2 poles (-1.9497, -12.3983) (-1.9497, -12.8614) (-2.3124, -13.6796) (-2.6675, -13.9806) knots 0 0 0 1 2 2 2
  spline S221 degree 2 poles (-2.6675, -13.9806) (-3.0457, -14.2971) (-4.0106, -14.629) (-4.7439, -14.629) knots 0 0 0 1 2 2 2
  line L151 (0.3969, -14.4592) -> (-0.8073, -14.4592)
  line L152 (-0.8073, -14.4592) -> (-0.8073, -7.3116)
  line L153 (-0.8073, -7.3116) -> (0.3969, -7.3116)
  line L154 (0.3969, -7.3116) -> (0.3969, -14.4592)
  line L155 (0.4818, -6.1229) -> (-0.8845, -6.1229)
  line L156 (-0.8845, -6.1229) -> (-0.8845, -4.8724)
  line L157 (-0.8845, -4.8724) -> (0.4818, -4.8724)
  line L158 (0.4818, -4.8724) -> (0.4818, -6.1229)
  spline S222 degree 2 poles (8.0385, -10.8854) (8.0385, -12.6916) (6.3017, -14.6599) (4.8506, -14.6599) knots 0 0 0 1 2 2 2
  spline S223 degree 2 poles (4.8506, -14.6599) (3.3609, -14.6599) (1.655, -12.6298) (1.655, -10.8854) knots 0 0 0 1 2 2 2
  spline S224 degree 2 poles (1.655, -10.8854) (1.655, -9.0946) (3.4149, -7.1109) (4.8506, -7.1109) knots 0 0 0 1 2 2 2
  spline S225 degree 2 poles (4.8506, -7.1109) (6.3017, -7.1109) (8.0385, -9.0869) (8.0385, -10.8854) knots 0 0 0 1 2 2 2
  spline S226 degree 2 poles (6.7957, -10.8854) (6.7957, -9.496) (5.7846, -8.1452) (4.8506, -8.1452) knots 0 0 0 1 2 2 2
  spline S227 degree 2 poles (4.8506, -8.1452) (3.9166, -8.1452) (2.8977, -9.496) (2.8977, -10.8854) knots 0 0 0 1 2 2 2
  spline S228 degree 2 poles (2.8977, -10.8854) (2.8977, -12.2362) (3.9166, -13.6256) (4.8506, -13.6256) knots 0 0 0 1 2 2 2
  spline S229 degree 2 poles (4.8506, -13.6256) (5.7769, -13.6256) (6.7957, -12.2593) (6.7957, -10.8854) knots 0 0 0 1 2 2 2
  line L159 (14.885, -14.4592) -> (13.6809, -14.4592)
  line L160 (13.6809, -14.4592) -> (13.6809, -10.3837)
  spline S230 degree 2 poles (13.6809, -10.3837) (13.6809, -9.8897) (13.5883, -9.0406) (13.4493, -8.7859) knots 0 0 0 1 2 2 2
  spline S231 degree 2 poles (13.4493, -8.7859) (13.3027, -8.5157) (12.7778, -8.2533) (12.3301, -8.2533) knots 0 0 0 1 2 2 2
  spline S232 degree 2 poles (12.3301, -8.2533) (11.8824, -8.2533) (10.933, -8.7318) (10.4776, -9.1178) knots 0 0 0 1 2 2 2
  line L161 (10.4776, -9.1178) -> (10.4776, -14.4592)
  line L162 (10.4776, -14.4592) -> (9.2735, -14.4592)
  line L163 (9.2735, -14.4592) -> (9.2735, -7.3116)
  line L164 (9.2735, -7.3116) -> (10.4776, -7.3116)
  line L165 (10.4776, -7.3116) -> (10.4776, -8.1066)
  spline S233 degree 2 poles (10.4776, -8.1066) (11.0179, -7.6203) (12.06, -7.1109) (12.6466, -7.1109) knots 0 0 0 1 2 2 2
  spline S234 degree 2 poles (12.6466, -7.1109) (13.6963, -7.1109) (14.885, -8.5003) (14.885, -9.8202) knots 0 0 0 1 2 2 2
  line L166 (14.885, -9.8202) -> (14.885, -14.4592)
  spline S235 degree 2 poles (26.4169, -9.6967) (26.4169, -12.2593) (24.9272, -14.6599) (23.3757, -14.6599) knots 0 0 0 1 2 2 2
  spline S236 degree 2 poles (23.3757, -14.6599) (21.8011, -14.6599) (20.3268, -12.213) (20.3268, -9.7044) knots 0 0 0 1 2 2 2
  spline S237 degree 2 poles (20.3268, -9.7044) (20.3268, -7.1263) (21.8165, -4.7412) (23.3757, -4.7412) knots 0 0 0 1 2 2 2
  spline S238 degree 2 poles (23.3757, -4.7412) (24.9426, -4.7412) (26.4169, -7.2112) (26.4169, -9.6967) knots 0 0 0 1 2 2 2
  spline S239 degree 2 poles (24.7805, -12.599) (24.9658, -12.1281) (25.1202, -10.677) (25.1202, -9.6967) knots 0 0 0 1 2 2 2
  spline S240 degree 2 poles (25.1202, -9.6967) (25.1202, -8.7164) (24.9658, -7.273) (24.7728, -6.7867) knots 0 0 0 1 2 2 2
  spline S241 degree 2 poles (24.7728, -6.7867) (24.5799, -6.3004) (23.9083, -5.7987) (23.3757, -5.7987) knots 0 0 0 1 2 2 2
  spline S242 degree 2 poles (23.3757, -5.7987) (22.8431, -5.7987) (22.1562, -6.3004) (21.9555, -6.8021) knots 0 0 0 1 2 2 2
  spline S243 degree 2 poles (21.9555, -6.8021) (21.7625, -7.2884) (21.6236, -8.7704) (21.6236, -9.7044) knots 0 0 0 1 2 2 2
  spline S244 degree 2 poles (21.6236, -9.7044) (21.6236, -10.7079) (21.7471, -12.0509) (21.9477, -12.5758) knots 0 0 0 1 2 2 2
  spline S245 degree 2 poles (21.9477, -12.5758) (22.133, -13.0698) (22.82, -13.6024) (23.3757, -13.6024) knots 0 0 0 1 2 2 2
  spline S246 degree 2 poles (23.3757, -13.6024) (23.9006, -13.6024) (24.5876, -13.1007) (24.7805, -12.599) knots 0 0 0 1 2 2 2
  line L167 (33.5105, -14.4592) -> (27.6365, -14.4592)
  line L168 (27.6365, -14.4592) -> (27.6365, -13.1084)
  spline S247 degree 2 poles (27.6365, -13.1084) (28.2694, -12.5141) (29.3964, -11.4103) (29.9367, -10.8159) knots 0 0 0 1 2 2 2
  spline S248 degree 2 poles (29.9367, -10.8159) (31.0251, -9.6195) (31.8201, -8.1838) (31.8201, -7.4196) knots 0 0 0 1 2 2 2
  spline S249 degree 2 poles (31.8201, -7.4196) (31.8201, -7.0183) (31.5731, -6.4162) (31.3492, -6.2232) knots 0 0 0 1 2 2 2
  spline S250 degree 2 poles (31.3492, -6.2232) (31.1254, -6.0303) (30.5388, -5.8373) (30.1837, -5.8373) knots 0 0 0 1 2 2 2
  spline S251 degree 2 poles (30.1837, -5.8373) (29.8441, -5.8373) (29.1494, -6.0071) (28.8329, -6.1383) knots 0 0 0 1 2 2 2
  spline S252 degree 2 poles (28.8329, -6.1383) (28.5628, -6.2464) (28.061, -6.5551) (27.9067, -6.6632) knots 0 0 0 1 2 2 2
  line L169 (27.9067, -6.6632) -> (27.8372, -6.6632)
  line L170 (27.8372, -6.6632) -> (27.8372, -5.3047)
  spline S253 degree 2 poles (27.8372, -5.3047) (28.2308, -5.1117) (29.6434, -4.7335) (30.2763, -4.7335) knots 0 0 0 1 2 2 2
  spline S254 degree 2 poles (30.2763, -4.7335) (31.6117, -4.7335) (33.1168, -6.146) (33.1168, -7.3502) knots 0 0 0 1 2 2 2
  spline S255 degree 2 poles (33.1168, -7.3502) (33.1168, -7.9137) (32.8544, -8.8553) (32.6228, -9.2567) knots 0 0 0 1 2 2 2
  spline S256 degree 2 poles (32.6228, -9.2567) (32.3913, -9.6735) (31.7197, -10.4917) (31.3492, -10.8854) knots 0 0 0 1 2 2 2
  spline S257 degree 2 poles (31.3492, -10.8854) (30.7472, -11.5415) (29.2729, -12.9463) (28.8329, -13.3554) knots 0 0 0 1 2 2 2
  line L171 (28.8329, -13.3554) -> (33.5105, -13.3554)
  line L172 (33.5105, -13.3554) -> (33.5105, -14.4592)
  constraints: 2 end point, 2 horizontal, 1 horizontal alignment, 1 other
extrude "Extrusion3" cut sketch "Sketch2" against normal blind 1.27
equation "\"d0\" = insideDiameter"
equation "\"d1\" = wallThickness"
equation "\"d2\" = topThickness"
equation "\"d4\" = supportThickness"
equation "\"d6\" = textDepth"
equation "\"insideDiameter\" = 174.625"
equation "\"wallThickness\" = 4.7625"
equation "\"topThickness\" = 4.7625"
equation "\"supportThickness\" = 31.75"
equation "\"textDepth\" = 1.27"
body "Solid1"
